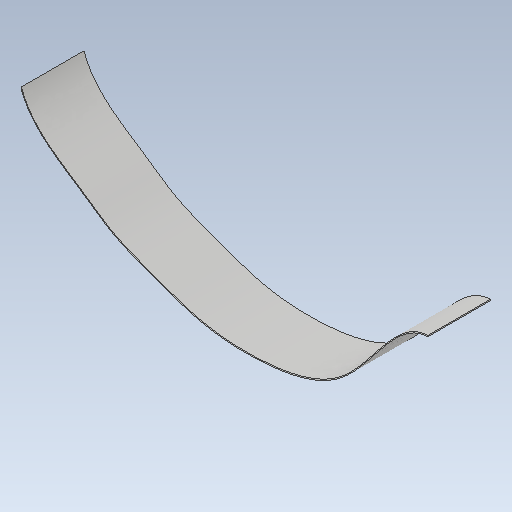
# Autodesk Inventor part: flexcable6
Saved by Autodesk Inventor 2020 (Build 240168000, 168)
## iProperties
Created: 2020-03-27
Part Number: flexcable6
Material: Generic
Document SubType Name: Modeling
Designer: Thomas Zhihao Luo
Density: 1 g/cm^3
Appearance: Default
Author: Thomas Zhihao Luo
Autodesk Inventor part; units mm, degrees
ref_plane "YZ Plane" through (0, 0, 0) normal (1, 0, 0) x (0, 1, 0)
ref_plane "XZ Plane" through (0, 0, 0) normal (0, 1, 0) x (-1, 0, 0)
ref_plane "XY Plane" through (0, 0, 0) normal (0, 0, 1) x (1, 0, 0)
sketch "Sketch1" plane through (0, 0, 0) normal (0, 0, 1) x (1, 0, 0)
  line L0 (45.4747, -6.1198) -> (45.4747, -6.0398) projected
  line L1 (17.55, -5.224) -> (17.55, -6.424) projected
  spline S0 degree 4 poles (17.55, -5.224) (18.1179, -6.9858) (20.2608, -8.3998) (21.7184, -9.2319) (24.0831, -11.0699) (27.3474, -12.0685) (29.8264, -13.2026) (34.2657, -13.4498) (39.6246, -12.3661) (41.4108, -9.7184) (43.5576, -6.0878) (45.4747, -6.0398) knots 0 0 0 0 0 0.200534 0.27813 0.360254 0.453696 0.554907 0.655457 0.758151 1 1 1 1 1
  spline S1 degree 4 poles (17.55, -5.3915) (18.1456, -7.07) (20.2684, -8.4898) (21.7242, -9.3161) (24.0831, -11.1511) (27.3475, -12.149) (29.8264, -13.2831) (34.2658, -13.5299) (39.6246, -12.4461) (41.4108, -9.7984) (43.5576, -6.1678) (45.4747, -6.1198) knots 0 0 0 0 0 0.199686 0.277363 0.359573 0.453114 0.554431 0.655089 0.757892 1 1 1 1 1
  point P0 (0, 0)
  point P1 (19.3337, -7.6566)
  point P2 (21, -8.8468)
  point P3 (22.2794, -9.7097)
  point P4 (23.9457, -10.7809)
  point P5 (26.8618, -11.9711)
  point P6 (29.8516, -12.937)
  point P7 (34.2372, -13.2242)
  point P8 (38.1093, -12.3282)
  point P9 (40.4897, -10.5431)
  point P10 (42.8701, -7.6566)
  point P11 (19.3337, -7.7381)
  point P12 (21, -8.9281)
  point P13 (22.2795, -9.7908)
  point P14 (23.9458, -10.8618)
  point P15 (26.8618, -12.0517)
  point P16 (29.8517, -13.0174)
  point P17 (34.2372, -13.3044)
  point P18 (38.1093, -12.4083)
  point P19 (40.4897, -10.6231)
  point P20 (42.8701, -7.7367)
  constraints: 1 point on line, 24 other
extrude "Extrusion1" add sketch "Sketch1" along normal mid plane 4.3
body "Solid1"
